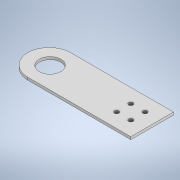
# Autodesk Inventor part: Beslag ekstra håndtag
Saved by Autodesk Inventor 2022 (Build 260153000, 153)
## iProperties
Created: 2022-04-12
Part Number: Beslag ekstra håndtag
Material: Generic
Document SubType Name: Sheet Metal
Designer: Patrick
Density: 1 g/cm^3
Sheet Metal Rule: Default_mm
Appearance: Default
Author: Patrick
Autodesk Inventor part; units mm, degrees
ref_plane "YZ Plane" through (0, 0, 0) normal (1, 0, 0) x (0, 1, 0)
ref_plane "XZ Plane" through (0, 0, 0) normal (0, 1, 0) x (-1, 0, 0)
ref_plane "XY Plane" through (0, 0, 0) normal (0, 0, 1) x (1, 0, 0)
sketch "Sketch1" plane through (0, 0, 0) normal (0, 1, 0) x (-1, 0, 0)
  line L0 (0, 0) -> (24, 0)
  line L1 (24, 0) -> (24, -24)
  line L2 (24, -24) -> (0, -24)
  line L3 (0, -24) -> (0, 0)
  circle A0 centre (57.5, -12) radius 6.1
  line L4 (24, 0) -> (70, 0)
  line L5 (70, 0) -> (70, -24)
  line L6 (70, -24) -> (24, -24)
  line L7 (24, -24) -> (24, 0)
  circle A1 centre (16, -16) radius 1.25
  circle A2 centre (8, -16) radius 1.25
  circle A3 centre (16, -8) radius 1.25
  circle A4 centre (8, -8) radius 1.25
  dimension "d0" = 24
  dimension "d1" = 24
  dimension "d6" = 12.2
  dimension "d20" = 12.5
  dimension "d21" = 12
  dimension "d22" = 46
  dimension "d23" = 2.5
  dimension "d24" = 8
  dimension "d25" = 8
  dimension "d28" = 8
  dimension "d31" = 8
  measures "d0" distance of L2.end L0.start
  measures "d1" distance of L1.end L2.end
  measures "d6" diameter of A0
  measures "d20" distance from line of L5 A0.centre
  measures "d21" distance from line of L4 A0.centre
  measures "d22" distance of L5.end L6.end
  measures "d23" diameter of A1
  measures "d24" distance from line of L2 A1.centre
  measures "d25" distance from line of L1 A1.centre
  measures "d28" distance of A1.centre A2.centre
  measures "d31" distance of A1.centre A3.centre
extrude "Plate2" add sketch "Sketch1" along normal blind 1.5
fillet "Fillet1" radius 12 2 edges at (-70, 0.75, 0) (-70, 0.75, -24)
equation "\"d34\" = Thickness"
equation "\"BendRadius\" = Thickness"
equation "\"BendReliefWidth\" = Thickness"
equation "\"BendReliefDepth\" = 0.5 * Thickness"
equation "\"CornerReliefSize\" = 4 * Thickness"
equation "\"MinimumRemnant\" = 2 * Thickness"
equation "\"TransitionRadius\" = BendRadius"
equation "\"JacobiRadiusSize\" = BendRadius"
equation "\"GapSize\" = Thickness"
equation "\"Thickness\" = 1.5"
body "Solid2"
